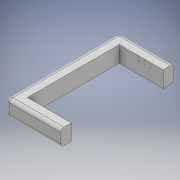
# Autodesk Inventor part: Bumper Side
Saved by Autodesk Inventor 2018 (Build 220112000, 112)
## iProperties
Created: 2020-01-22
Part Number: Bumper Side
Material: Generic
Document SubType Name: Modeling
Designer: s-2512711
Density: 1 g/cm^3
Appearance: Default
Author: s-2512711
Autodesk Inventor part; units mm, degrees
ref_plane "YZ Plane" through (0, 0, 0) normal (1, 0, 0) x (0, 1, 0)
ref_plane "XZ Plane" through (0, 0, 0) normal (0, 1, 0) x (-1, 0, 0)
ref_plane "XY Plane" through (0, 0, 0) normal (0, 0, 1) x (1, 0, 0)
sketch "Sketch1" plane through (0, 0, 0) normal (0, 0, 1) x (1, 0, 0)
  line L0 (0, 0) -> (0, 719.074)
  line L1 (0, 719.074) -> (342.9, 719.074)
  line L2 (0, 0) -> (342.9, 0)
  line L3 (342.9, 801.624) -> (-82.55, 801.624)
  line L4 (-82.55, 801.624) -> (-82.55, -82.55)
  line L5 (-82.55, -82.55) -> (342.9, -82.55)
  line L6 (342.9, 719.074) -> (342.9, 801.624)
  line L7 (342.9, 0) -> (342.9, -82.55)
  dimension "d0" = 719.074
  dimension "d1" = 342.9
  dimension "d2" = 82.55
  constraints: 16 end point, 2 perpendicular, 2 vertical, 1 collinear, 1 horizontal, 2 other
  measures "d0" distance of L0.start L0.end
  measures "d1" distance of L0.end L1.end
  measures "d2" distance between parallel lines of L0 L4
extrude "Extrusion1" add sketch "Sketch1" along normal blind 127
fillet "Fillet1" radius 25.4 8 edges at (130.175, 801.624, 127) (130.175, 801.624, 0) (-82.55, 801.624, 63.5) (-82.55, 359.537, 127) (-82.55, 359.537, 0) (-82.55, -82.55, 63.5) (130.175, -82.55, 0) (130.175, -82.55, 127)
sketch "Sketch2" plane through (0, 719.074, 0) normal (0, -1, 0) x (1, 0, 0)
  line L0 (342.9, 0) -> (342.9, 127) construction
  line L1 (0, 127) -> (342.9, 127) construction
  line L2 (342.9, 127) -> (241.3, 127) construction
  line L3 (241.3, 127) -> (196.85, 127) construction
  line L4 (196.85, 127) -> (152.4, 127) construction
  line L5 (241.3, 127) -> (241.3, 117.475) construction
  line L6 (241.3, 117.475) -> (196.85, 117.475) construction
  line L7 (196.85, 117.475) -> (152.4, 117.475) construction
  line L8 (152.4, 117.475) -> (152.4, 92.075) construction
  line L9 (152.4, 92.075) -> (196.85, 92.075) construction
  line L10 (196.85, 92.075) -> (241.3, 92.075) construction
  circle A0 centre (241.3, 117.475) radius 2.667
  circle A1 centre (196.85, 117.475) radius 2.667
  circle A2 centre (152.4, 117.475) radius 2.667
  circle A3 centre (152.4, 92.075) radius 2.667
  circle A4 centre (196.85, 92.075) radius 2.667
  circle A5 centre (241.3, 92.075) radius 2.667
  point P0 (0, 0)
  dimension "d7" = 101.6
  dimension "d8" = 44.45
  dimension "d9" = 44.45
  dimension "d10" = 9.525
  dimension "d11" = 25.4
  dimension "d12" = 5.334
  constraints: 18 end point, 6 centre point, 6 coincident, 6 point on line, 3 perpendicular, 1 vertical
  measures "d7" distance of L0.end L2.end
  measures "d8" distance of L2.end L3.end
  measures "d9" distance of L3.end L4.end
  measures "d10" distance of L2.end L5.end
  measures "d11" distance of L7.end L8.end
  measures "d12" diameter of A0
extrude "Extrusion2" cut sketch "Sketch2" against normal blind 4.7625
sketch "Sketch3" plane through (0, 0, 0) normal (0, 1, 0) x (1, 0, 0)
  line L0 (342.9, -127) -> (0, -127) construction
  line L1 (342.9, -127) -> (342.9, -117.475) construction
  line L2 (342.9, 0) -> (342.9, -127) construction
  line L3 (342.9, -117.475) -> (241.3, -117.475) construction
  line L4 (241.3, -117.475) -> (196.85, -117.475) construction
  line L5 (196.85, -117.475) -> (152.4, -117.475) construction
  line L6 (152.4, -117.475) -> (152.4, -92.075) construction
  line L7 (152.4, -92.075) -> (196.85, -92.075) construction
  line L8 (196.85, -92.075) -> (241.3, -92.075) construction
  circle A0 centre (241.3, -117.475) radius 2.667
  circle A1 centre (196.85, -117.475) radius 2.667
  circle A2 centre (152.4, -117.475) radius 2.667
  circle A3 centre (152.4, -92.075) radius 2.667
  circle A4 centre (196.85, -92.075) radius 2.667
  circle A5 centre (241.3, -92.075) radius 2.667
  point P0 (0, 0)
  dimension "d15" = 9.525
  dimension "d16" = 101.6
  dimension "d17" = 44.45
  dimension "d18" = 44.45
  dimension "d19" = 25.4
  dimension "d20" = 5.334
  constraints: 14 end point, 6 centre point, 6 coincident, 3 point on line, 2 horizontal, 2 perpendicular
  measures "d15" distance of L0.start L1.end
  measures "d16" distance of L1.end L3.end
  measures "d17" distance of L3.end L4.end
  measures "d18" distance of L4.end L5.end
  measures "d19" distance of L5.end L6.end
  measures "d20" diameter of A0
extrude "Extrusion3" cut sketch "Sketch3" against normal blind 4.7625
body "Solid1"
